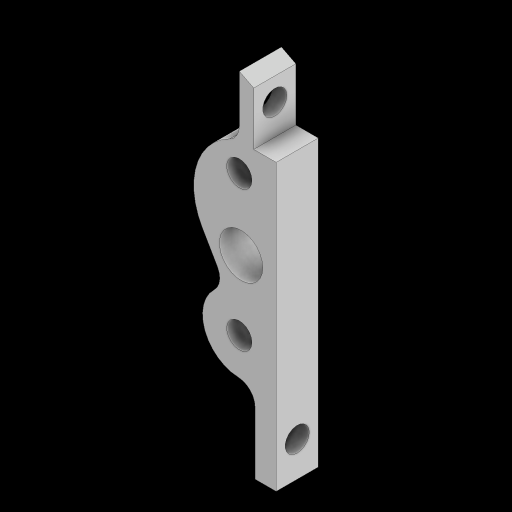
# Autodesk Inventor part: DrivenMotorMount
Saved by Autodesk Inventor 2024.1 (Build 281209000, 209)
## iProperties
Created: 2025-05-07
Part Number: DrivenMotorMount
Material: Generic
Document SubType Name: Modeling
Designer: Teddy
Density: 1 g/cm^3
Appearance: Default
Author: Teddy
Autodesk Inventor part; units mm, degrees
ref_plane "YZ Plane" through (0, 0, 0) normal (1, 0, 0) x (0, 1, 0)
ref_plane "Work Plane1" through (0, 0, 0) normal (0, 0, 1) x (1, 0, 0)
ref_plane "Work Plane2" through (-23.495, -37.0586, -7.62) normal (0, 0, -1) x (0, 1, 0)
sketch "Sketch1" plane through (0, 0, 0) normal (0, 0, 1) x (1, 0, 0)
  circle A0 centre (-14.605, 0) radius 3.81
  line L0 (23.495, -13.6398) -> (23.495, -75.1078)
  line L1 (-14.605, 0) -> (17.145, -54.9926) construction
  circle A1 centre (17.145, -54.9926) radius 3.937
  line L2 (-14.605, 0) -> (17.145, 54.9926) construction
  circle A2 centre (17.145, 54.9926) radius 2.286
  line L3 (19.685, -33.9344) -> (23.495, -33.9344)
  line L4 (19.685, -29.5656) -> (23.495, -29.5656)
  line L5 (23.495, -46.7614) -> (25.0825, -46.7614)
  line L6 (23.495, -72.1614) -> (25.0825, -72.1614)
  line L7 (23.495, -67.5386) -> (25.0825, -67.5386)
  line L8 (23.495, -76.1238) -> (25.0825, -76.1238)
  line L9 (10.1391, -54.1676) -> (16.832, -37.0586)
  line L10 (16.832, -37.0586) -> (16.832, -26.036)
  line L11 (19.685, -27.493) -> (-18.6482, -7.9174)
  line L12 (19.685, -27.493) -> (19.685, -37.0586)
  line L13 (19.685, -37.0586) -> (23.495, -37.0586)
  line L14 (23.495, -37.0586) -> (23.495, -64.1344)
  line L15 (23.495, -64.1344) -> (15.875, -64.1344)
  line L16 (19.685, -64.1344) -> (19.685, -76.1238)
  line L17 (19.685, -76.1238) -> (23.495, -76.1238)
  line L18 (15.875, -64.1344) -> (10.1391, -54.1676)
  line L19 (19.431, -27.3632) -> (19.431, -37.0586)
  line L20 (19.431, -37.0586) -> (19.685, -37.0586)
  line L21 (16.832, -26.2966) -> (19.685, -27.7535)
  line L22 (19.431, -37.0586) -> (19.431, -37.241)
  line L23 (19.431, -37.241) -> (23.495, -37.241)
  line L24 (23.495, -76.1238) -> (23.495, -64.1344)
  circle A3 centre (16.832, -42.2926) radius 2.286
  circle A4 centre (16.832, -67.6926) radius 2.286
  arc A5 (16.832, -37.0586) -> (10.1391, -54.1676) centre (20.3426, -48.2955) ccw
  circle A6 centre (16.832, -67.6926) radius 6.6647
  line L25 (16.832, -74.3574) -> (23.495, -74.3574)
  line L26 (23.495, -76.1238) -> (23.495, -88.8238)
  line L27 (23.495, -88.8238) -> (19.685, -88.8238)
  line L28 (19.685, -88.8238) -> (19.685, -76.1238)
  point P0 (0, 0)
  point P1 (23.495, -37.241)
  point P2 (19.431, -27.6238)
  point P3 (14.3606, -61.503)
  point P4 (19.685, -74.3574)
extrude "Extrusion1" add sketch "Sketch1" against normal up to surface (7.62 mm away) contours L0 L15 A6 L18 L9 A3 L10 L21 L19 L22 L23 | L0 A6 L15 | L9 A3 A5 | L0 A6 L16 L15 | L15 L18 A6 | L0 L25 L16 A6 | L16 A6 L18 L15 | L16 L25 A6 | L0 L24 L17 L16 L25 | L17 L26 L27 L28
sketch "Sketch2" plane through (19.685, -76.1238, 0) normal (-1, 0, 0) x (0, 0, 1)
  circle A0 centre (-3.81, 6.2738) radius 2.1844 projected
  circle A1 centre (-3.81, 44.3738) radius 2.1844 projected
  circle A2 centre (-3.81, 44.3738) radius 2.1844 projected
  circle A3 centre (-3.81, -6.4262) radius 2.1844
  point P0 (0, 76.1238)
  dimension "d22" = 50.8
  constraints: 1 centre point, 1 equal radius
  measures "d22" distance of A1.centre A3.centre
extrude "Extrusion2" cut sketch "Sketch2" along normal mid plane 25.4 contours A1 | A3
fillet "Fillet1" radius 3.175 2 edges at (14.3606, -61.503, -3.81) (16.832, -37.0586, -3.81)
fillet "Fillet2" radius 3.175 1 edges at (19.685, -74.3574, -3.81)
body "Solid1"
